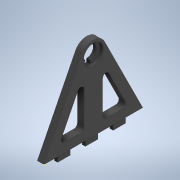
# Autodesk Inventor part: spool holder arm
Saved by Autodesk Inventor 2020.2 (Build 242310000, 310)
## iProperties
Created: 2020-02-07
Part Number: spool holder arm
Material: PLA
Document SubType Name: Modeling
Designer: mulve
Density: 1.3 g/cm^3
Appearance: Generic
Mass: 104.62 g
Surface Area: 258.571 cm^2
Volume: 80.4765 cm^3
Author: mulve
Autodesk Inventor part; units mm, degrees
ref_plane "YZ Plane" through (0, 0, 0) normal (1, 0, 0) x (0, 1, 0)
ref_plane "XZ Plane" through (0, 0, 0) normal (0, 1, 0) x (-1, 0, 0)
ref_plane "XY Plane" through (0, 0, 0) normal (0, 0, 1) x (1, 0, 0)
sketch "Sketch1" plane through (0, 0, 0) normal (1, 0, 0) x (0, 1, 0)
  line L0 (150, -75) -> (0, 0)
  line L1 (150, -75) -> (0, -150)
  line L2 (0, -150) -> (0, 0)
  dimension "d0" = 150
  dimension "d1" = 75
  constraints: 6 end point, 1 equal length, 1 vertical
  measures "d0" horizontal distance of L0.end L0.start
  measures "d1" vertical distance of L0.end L0.start
extrude "Extrusion1" add sketch "Sketch1" along normal blind 10.16
sketch "Sketch2" plane through (10.16, 0, 0) normal (1, 0, 0) x (0, 0, -1)
  point P0 (0, 0)
fillet "Fillet1" radius 19.05 1 edges at (5.08, 150, -75)
sketch "Sketch3" plane through (10.16, 0, 0) normal (1, 0, 0) x (0, 0, -1)
  arc A0 (92.0388, 115.9223) -> (57.9612, 115.9223) centre (75, 107.4029) ccw projected
  circle A1 centre (75, 107.4029) radius 15
  circle A2 centre (75, 107.4029) radius 10
  line L0 (75, 122.4029) -> (75, 117.4029)
  line L1 (75, 97.4029) -> (75, 92.4029)
  line L2 (85.6066, 118.0095) -> (82.0711, 114.474)
  line L3 (67.9289, 100.3318) -> (64.3934, 96.7963)
  point P0 (0, 0)
  dimension "d5" = 30
  dimension "d34" = 20
  dimension "d35" = 45
  dimension "d36" = 45
  constraints: 8 end point, 8 line through centre, 8 point on circle, 2 centre point, 2 coincident, 2 point on line, 1 vertical
  measures "d5" diameter of A1
  measures "d34" diameter of A2
  measures "d35" angle of L2 L0
  measures "d36" angle of L1 L3
sketch "Sketch4" plane through (10.16, 0, 0) normal (1, 0, 0) x (0, 0, -1)
  line L0 (22.8055, 14.0945) -> (60.9055, 90.2945)
  line L1 (57.9612, 115.9223) -> (0, 0) projected
  line L2 (22.8055, 14.0945) -> (60.9055, 14.0945)
  line L3 (60.9055, 14.0945) -> (60.9055, 90.2945)
  line L4 (0, 0) -> (150, 0) construction
  line L5 (0, 0) -> (150, 0) construction
  arc A0 (92.0388, 115.9223) -> (57.9612, 115.9223) centre (75, 107.4029) ccw construction
  line L6 (75, 126.4529) -> (75, 0) construction
  line L7 (127.1945, 14.0945) -> (89.0945, 90.2945)
  line L8 (127.1945, 14.0945) -> (89.0945, 14.0945)
  line L9 (89.0945, 14.0945) -> (89.0945, 90.2945)
  dimension "d8" = 76.2
  dimension "d11" = 14.0945
  dimension "d12" = 14.0945
  dimension "d13" = 14.0945
  constraints: 16 end point, 3 symmetric about line, 2 horizontal, 1 midpoint, 1 parallel, 1 perpendicular, 1 point on circle
  measures "d8" distance of L2.end L0.end
  measures "d11" distance between parallel lines of L6 L3
  measures "d12" distance between parallel lines of L4 L2
  measures "d13" distance between parallel lines of L1 L0
extrude "Extrusion3" cut sketch "Sketch4" against normal through all
fillet "Fillet2" radius 5 1 edges at (5.08, 14.0945, -127.1945)
fillet "Fillet3" radius 5 2 edges at (5.08, 14.0945, -89.0945) (5.08, 90.2945, -89.0945)
fillet "Fillet4" radius 5 3 edges at (5.08, 14.0945, -60.9055) (5.08, 90.2945, -60.9055) (5.08, 14.0945, -22.8055)
sketch "Sketch6" plane through (0, 0, -150) normal (0, -1, 0) x (1, 0, 0)
  line L0 (10.16, 150) -> (10.16, 0) construction
  line L1 (10.16, 75) -> (0, 75) construction
  line L2 (0, 65) -> (0, 85) construction
  line L3 (7.493, 126.597) -> (2.667, 126.597)
  line L4 (2.667, 126.597) -> (2.667, 107.801)
  line L5 (2.667, 107.801) -> (7.493, 107.801)
  line L6 (7.493, 107.801) -> (7.493, 126.597)
  line L7 (0, 150) -> (0, 0) projected
  line L8 (0, 150) -> (10.16, 150) projected
  line L9 (7.493, 84.398) -> (2.667, 84.398)
  line L10 (2.667, 84.398) -> (2.667, 65.602)
  line L11 (2.667, 65.602) -> (7.493, 65.602)
  line L12 (7.493, 65.602) -> (7.493, 84.398)
  line L13 (7.493, 23.403) -> (2.667, 23.403)
  line L14 (2.667, 23.403) -> (2.667, 42.199)
  line L15 (2.667, 42.199) -> (7.493, 42.199)
  line L16 (7.493, 42.199) -> (7.493, 23.403)
  dimension "d22" = 4.826
  dimension "d23" = 2.667
  dimension "d24" = 2.667
  dimension "d25" = 18.796
  dimension "d26" = 23.403
  dimension "d27" = 18.796
  dimension "d29" = 4.826
  dimension "d30" = 2.667
  dimension "d31" = 2.667
  dimension "d41" = 23.403
  constraints: 26 end point, 4 parallel, 4 symmetric about line, 2 horizontal, 2 midpoint, 2 perpendicular, 1 other
  measures "d22" distance of L4.end L5.end
  measures "d23" distance between parallel lines of L0 L6
  measures "d24" distance between parallel lines of L7 L4
  measures "d25" distance of L5.end L3.start
  measures "d26" distance between parallel lines of L8 L3
  measures "d27" distance of L11.end L9.start
  measures "d29" distance of L9.start L9.end
  measures "d30" distance between parallel lines of L0 L12
  measures "d31" distance between parallel lines of L2 L10
  measures "d41" distance between parallel lines of L5 L9
extrude "Extrusion5" add sketch "Sketch6" along normal blind 10.16
extrude "Extrusion6" cut sketch "Sketch3" against normal through all contours L2 A2 L0 A1 | A1 L3 A2 L1 | A2
extrude "Extrusion7" cut sketch "Sketch3" against normal blind 5.08 contours A1 L1 A2 L2 | L0 A2 L3 A1
equation "\"d11\" = d13"
equation "\"d12\" = d11"
equation "\"d23\" = d24"
equation "\"d26\" = d41"
equation "\"d27\" = d25"
equation "\"d29\" = d22"
equation "\"d30\" = d23"
body "Solid1"
